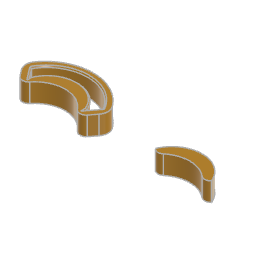
snout-spacer v8 (Autodesk Fusion 360 design; units mm, degrees)
Autodesk Fusion 360 part; units mm, degrees
sketch "Sketch1" plane through (0, 0, 0) normal (0, 0, 1) x (1, 0, 0)
  line L0 (0, 0) -> (9, 0) construction
  line L1 (0, -2) -> (9, -2) construction
  line L2 (4.5, 0) -> (4.5, 1) construction
  arc A0 (9, -2) -> (0, -2) centre (4.5, -3.875) ccw
  line L3 (4.5, 0) -> (4.5, 3) construction
  arc A1 (9, 0) -> (0, 0) centre (4.5, -1.875) ccw
  line L4 (9, -2) -> (9, 0)
  line L5 (0, -2) -> (0, 0)
  line L6 (-1.0113, 1.318) -> (10.0114, 1.318) construction
  line L7 (9, 0) -> (10.0114, 1.318) construction
  line L8 (0, 0) -> (-1.0113, 1.318) construction
  line L9 (4.5, 1.318) -> (4.5, 4.5) construction
  arc A2 (10.0114, 1.318) -> (-1.0113, 1.318) centre (4.5, -1.8639) ccw construction
  line L10 (0, -0.2464) -> (-1.1304, 1.2267)
  line L11 (9, -0.2464) -> (10.1304, 1.2267)
  line L12 (-1.1304, 1.2267) -> (-1.0113, 1.318) construction
  line L13 (-1.1304, 1.2267) -> (-1.2217, 1.3457)
  line L14 (10.1304, 1.2267) -> (10.2217, 1.3457)
  arc A3 (10.2217, 1.3457) -> (-1.2217, 1.3457) centre (4.5, -1.9559) ccw
  line L15 (4.5, 4.5) -> (4.5, 4.65) construction
  line L16 (0, -2) -> (-2.4351, 1.1734)
  line L17 (9, -2) -> (11.4351, 1.1734)
  arc A4 (11.4351, 1.1734) -> (-2.4351, 1.1734) centre (4.5, -2.2214) ccw
  dimension "d1" = 9
  dimension "d2" = 9
  dimension "d3" = 2
  dimension "d4" = 1
  dimension "d5" = 3
  dimension "d8" = 11.0227
  dimension "d10" = 1.318
  dimension "d13" = 0.15
  dimension "d14" = 3.182
  dimension "d15" = 0.15
  dimension "d16" = 0.15
  dimension "d17" = 0.15
  dimension "d18" = 4
  constraint coincident L0.start A1.end
  constraint horizontal L0
  constraint horizontal L1
  constraint midpoint L0 L2.start
  constraint perpendicular L0 L2
  constraint coincident L2.end A0
  constraint perpendicular L0 L3
  constraint coincident L3.end A1
  constraint perpendicular L0 L4
  constraint parallel L0 L6
  constraint midpoint L6 L9.start
  constraint perpendicular L6 L9
  constraint coincident L9.end A2
  constraint coincident L5 L10.start
  constraint parallel L8 L10
  constraint collinear L3 L9
  constraint symmetric L9 L10.start L11.start
  constraint symmetric L9 L10.end L11.end
  constraint coincident L8 L6.start
  constraint perpendicular L8 L12
  constraint coincident L6.start L12
  constraint perpendicular L12 L13
  constraint parallel L11 L14
  constraint midpoint A3 L15.end
  constraint parallel L10 L16
  constraint symmetric L1.start L9 L1.end
  constraint symmetric L9 L16.end L17.end
  measures "d1" distance of L0.start L0.end
  measures "d2" distance of L1.start L1.end
  measures "d3" distance of L0 L1
  measures "d4" distance of L2.start L2.end
  measures "d5" distance of L2.start L3.end
  measures "d8" distance of L6.start L6.end
  measures "d10" distance of L0 L6
  measures "d13" distance of L8 L10
  measures "d14" distance of L9.start L9.end
  measures "d15" distance of L10.end L13.end
  measures "d16" distance of L11.end L14.end
  measures "d17" distance of L9.end L15.end
  measures "d18" distance of L1.start L16.end
extrude "Extrude1" add sketch "Sketch1" along normal blind 3 contours A0 A1 L4 L5 makes body 1
copy_body "CopyPasteBodies1" bodies 1 makes body 2
move_body "Move1" bodies 2 to x (1, 0, 0) y (0, 1, 0) z (0, 0, 1) at (20, 0, 0)
extrude "Extrude2" add sketch "Sketch1" along normal up to surface (3 mm away) contours L4 L5 L10 L11 L13 L14 A3 L16 L17 A4 bodies 1
fillet "Fillet1" radius 1.75 2 edges at (-2.4351, 1.1734, 1.5) (11.4351, 1.1734, 1.5) on bodies 1
chamfer "Chamfer1" distance 0.2 angle 45 6 edges at (4.5, 3, 3) (9, -0.1232, 3) (9.6108, 0.5496, 3) (4.5, 4.65, 3) (0, -0.1232, 3) (-0.6108, 0.5496, 3) on bodies 1
copy_body "Body->Comp1" bodies 2 removing the originals makes body 3 in component "snout-spacer"
copy_body "Body->Comp2" bodies 1 removing the originals makes body 4 in component "snout-spacer self-fit"
fillet "Fillet1'" radius 1 2 edges at (20, -2, 1.5) (29, -2, 1.5) on bodies 3 in component "snout-spacer"
fillet "Fillet1''" radius 1 2 edges at (9, -2, 1.5) (0, -2, 1.5) on bodies 4 in component "snout-spacer self-fit"
component "snout-spacer" placed x (1, 0, 0) y (0, 1, 0) z (0, 0, 1) at (0, 0, 0)
component "snout-spacer self-fit" placed x (1, 0, 0) y (0, 1, 0) z (0, 0, 1) at (0, 0, 0)
